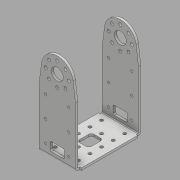
# Autodesk Inventor part: f4Bracket
Saved by Autodesk Inventor 2017.3 (Build 213257000, 257)
## iProperties
Created: 2020-01-31
Part Number: f4Bracket
Material: Generic
Document SubType Name: Modeling
Designer: Tirza Sarwono
Density: 1 g/cm^3
Appearance: Default
Author: Tirza Sarwono
Autodesk Inventor part; units mm, degrees
ref_plane "YZ Plane" through (0, 0, 0) normal (1, 0, 0) x (0, 1, 0)
sketch "Sketch5" plane through (0, 0, 0) normal (0, 0, 1) x (1, 0, 0)
  line L0 (0, 0) -> (25, 0)
  line L1 (25, 1) -> (25, 0)
  line L2 (25, 1) -> (26, 1)
  line L3 (26, 1) -> (26, 40)
  line L4 (26, 40) -> (25, 40)
  line L5 (25, 41) -> (25, 40)
  line L6 (25, 41) -> (0, 41)
  line L7 (0, 40) -> (0, 41)
  line L8 (0, 40) -> (-1, 40)
  line L9 (-1, 40) -> (-1, 1)
  line L10 (-1, 1) -> (0, 1)
  line L11 (0, 0) -> (0, 1)
  line L12 (10.4003, 25.5003) -> (14.6003, 25.5003)
  arc A0 (16.6003, 23.5003) -> (14.6003, 25.5003) centre (14.6003, 23.5003) ccw
  line L13 (16.6003, 23.5003) -> (16.6003, 17.4997)
  arc A1 (14.6003, 15.4997) -> (16.6003, 17.4997) centre (14.6003, 17.4997) ccw
  line L14 (14.6003, 15.4997) -> (10.4003, 15.4997)
  arc A2 (8.4003, 17.4997) -> (10.4003, 15.4997) centre (10.4003, 17.4997) ccw
  line L15 (8.4003, 17.4997) -> (8.4003, 23.5003)
  arc A3 (10.4003, 25.5003) -> (8.4003, 23.5003) centre (10.4003, 23.5003) ccw
  circle A4 centre (4.5003, 12.5) radius 1.05
  circle A5 centre (4.5003, 20.5) radius 1.05
  circle A6 centre (4.5003, 28.5) radius 1.05
  circle A7 centre (20.5003, 4.5) radius 1.05
  circle A8 centre (4.5003, 4.5) radius 1.05
  circle A9 centre (4.5003, 36.5) radius 1.05
  circle A10 centre (20.5003, 36.5) radius 1.05
  circle A11 centre (20.5003, 20.5) radius 1.05
  circle A12 centre (12.5003, 12.5) radius 1.05
  circle A13 centre (12.5003, 28.5) radius 1.05
  circle A14 centre (20.5003, 12.5) radius 1.05
  circle A15 centre (20.5003, 28.5) radius 1.05
  point P0 (12.5003, 20.5)
  constraints: 32 end point, 16 centre point, 8 point on circle
extrude "Extrusion3" add sketch "Sketch5" along normal blind 1.588
sketch "Sketch6" plane through (0, 40, 0) normal (-1, 0, 0) x (0, 0, 1)
  line L0 (2.088, -40.5) -> (2.088, -42.0875)
  arc A0 (1.588, -40) -> (2.088, -40.5) centre (2.088, -40) ccw
  line L1 (0.0005, -40) -> (1.588, -40)
  arc A1 (0.0005, -40) -> (2.088, -42.0875) centre (2.088, -40) ccw
  line L2 (2.088, 3.0875) -> (2.088, 1.5)
  arc A2 (2.088, 3.0875) -> (0.0005, 1) centre (2.088, 1) ccw
  line L3 (1.588, 1) -> (0.0005, 1)
  arc A3 (2.088, 1.5) -> (1.588, 1) centre (2.088, 1) ccw
  point P0 (0, -40)
  point P1 (10.9999, -21)
  constraints: 8 end point, 8 point on circle, 4 centre point
extrude "Extrusion4" add sketch "Sketch6" against normal blind 25
ref_plane "Work Plane1" through (0, -2.0875, 2.088) normal (0, -1, 0) x (1, 0, 0)
sketch "Sketch7" plane through (0, -2.0875, 2.088) normal (0, -1, 0) x (1, 0, 0)
  line L0 (25, 39.4126) -> (23.406, 51.8112)
  arc A0 (23.406, 51.8112) -> (1.5893, 51.8033) centre (12.4982, 50.3905) ccw
  line L1 (1.5893, 51.8033) -> (0, 39.4048)
  line L2 (0, 39.4048) -> (0, 0)
  line L3 (0, 0) -> (25, 0)
  line L4 (25, 39.4126) -> (25, 0)
  circle A1 centre (12.5, 50.4125) radius 4.1
  circle A2 centre (20.5, 19.7062) radius 0.7835
  circle A3 centre (4.5, 19.7062) radius 0.7835
  circle A4 centre (20.5, 5) radius 0.7835
  circle A5 centre (20.5, 34.4125) radius 0.7835
  circle A6 centre (4.5, 34.4125) radius 0.7835
  circle A7 centre (4.5, 5) radius 0.7835
  circle A8 centre (18.1569, 56.0694) radius 1.05
  circle A9 centre (18.1569, 44.7556) radius 1.05
  circle A10 centre (6.8431, 44.7556) radius 1.05
  circle A11 centre (6.8431, 56.0694) radius 1.05
  circle A12 centre (4.5, 50.4125) radius 1.05
  circle A13 centre (20.5, 50.4125) radius 1.05
  circle A14 centre (12.5, 42.4125) radius 1.05
  circle A15 centre (12.5, 58.4125) radius 1.05
  arc A16 (7.5, 3) -> (8.5, 2) centre (8.5, 3) ccw
  line L5 (7.5, 3) -> (7.5, 7)
  arc A17 (8.5, 8) -> (7.5, 7) centre (8.5, 7) ccw
  line L6 (8.5, 8) -> (16.5, 8)
  arc A18 (17.5, 7) -> (16.5, 8) centre (16.5, 7) ccw
  line L7 (17.5, 7) -> (17.5, 3)
  arc A19 (16.5, 2) -> (17.5, 3) centre (16.5, 3) ccw
  line L8 (16.5, 2) -> (8.5, 2)
  point P0 (0, -2.088)
  point P1 (12.4997, 50.4125)
  constraints: 20 centre point, 18 end point, 10 point on circle
extrude "Extrusion5" add sketch "Sketch7" against normal blind 1.588
ref_plane "Work Plane2" through (0, 43.0875, 2.088) normal (0, -1, 0) x (1, 0, 0)
sketch "Sketch8" plane through (0, 43.0875, 2.088) normal (0, -1, 0) x (1, 0, 0)
  line L0 (25, 39.4126) -> (23.406, 51.8112)
  arc A0 (23.406, 51.8112) -> (1.5893, 51.8033) centre (12.4982, 50.3905) ccw
  line L1 (1.5893, 51.8033) -> (0, 39.4048)
  line L2 (0, 39.4048) -> (0, 0)
  line L3 (0, 0) -> (25, 0)
  line L4 (25, 39.4126) -> (25, 0)
  circle A1 centre (12.5, 50.4125) radius 4.1
  circle A2 centre (20.5, 19.7062) radius 0.7835
  circle A3 centre (4.5, 19.7062) radius 0.7835
  circle A4 centre (20.5, 5) radius 0.7835
  circle A5 centre (20.5, 34.4125) radius 0.7835
  circle A6 centre (4.5, 34.4125) radius 0.7835
  circle A7 centre (4.5, 5) radius 0.7835
  circle A8 centre (18.1569, 56.0694) radius 1.05
  circle A9 centre (18.1569, 44.7556) radius 1.05
  circle A10 centre (6.8431, 44.7556) radius 1.05
  circle A11 centre (6.8431, 56.0694) radius 1.05
  circle A12 centre (4.5, 50.4125) radius 1.05
  circle A13 centre (20.5, 50.4125) radius 1.05
  circle A14 centre (12.5, 42.4125) radius 1.05
  circle A15 centre (12.5, 58.4125) radius 1.05
  arc A16 (7.5, 3) -> (8.5, 2) centre (8.5, 3) ccw
  line L5 (7.5, 3) -> (7.5, 7)
  arc A17 (8.5, 8) -> (7.5, 7) centre (8.5, 7) ccw
  line L6 (8.5, 8) -> (16.5, 8)
  arc A18 (17.5, 7) -> (16.5, 8) centre (16.5, 7) ccw
  line L7 (17.5, 7) -> (17.5, 3)
  arc A19 (16.5, 2) -> (17.5, 3) centre (16.5, 3) ccw
  line L8 (16.5, 2) -> (8.5, 2)
  point P0 (0, -2.088)
  point P1 (12.4997, 50.4125)
  constraints: 20 centre point, 18 end point, 10 point on circle
extrude "Extrusion6" add sketch "Sketch8" along normal blind 1.588
body "Solid3"
